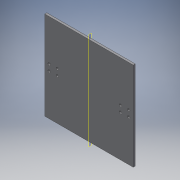
# Autodesk Inventor part: Hotplate
Saved by Autodesk Inventor 2019 (Build 230136000, 136)
## iProperties
Created: 2018-10-03
Part Number: Hotplate
Material: Generic
Document SubType Name: Modeling
Designer: LillaHunden
Mass: 231.125 g
Surface Area: 967.5 cm^2
Volume: 231.125 cm^3
Density: 1 g/cm^3
Appearance: Default
Author: LillaHunden
Autodesk Inventor part; units mm, degrees
ref_plane "YZ Plane" through (0, 0, 0) normal (1, 0, 0) x (0, 1, 0)
ref_plane "XZ Plane" through (0, 0, 0) normal (0, 1, 0) x (-1, 0, 0)
ref_plane "XY Plane" through (0, 0, 0) normal (0, 0, 1) x (1, 0, 0)
sketch "Sketch1" plane through (0, 0, 0) normal (0, 0, 1) x (1, 0, 0)
  line L0 (-107.5, -107.5) -> (107.5, -107.5)
  line L1 (107.5, -107.5) -> (107.5, 107.5)
  line L2 (107.5, 107.5) -> (-107.5, 107.5)
  line L3 (-107.5, 107.5) -> (-107.5, -107.5)
  line L4 (-107.5, -107.5) -> (107.5, 107.5) construction
  line L5 (107.5, -107.5) -> (-107.5, 107.5) construction
  point P0 (0, 0)
  dimension "d0" = 215
  dimension "d1" = 215
  constraints: 12 end point, 2 midpoint, 2 parallel, 1 horizontal, 1 perpendicular
  measures "d0" distance of L2.end L1.end
  measures "d1" distance of L1.end L0.end
extrude "Extrusion1" add sketch "Sketch1" along normal blind 5
ref_plane "Work Plane1" through (0, -107.5, 0) normal (-1, 0, 0) x (0, 0, 1)
sketch "Sketch3" plane through (0, 0, 5) normal (0, 0, 1) x (1, 0, 0)
  point P0 (96.652, 7.5)
  point P1 (96.652, -7.5)
  point P2 (76.652, -7.5)
  point P3 (76.652, 7.5)
  point P4 (-96.652, 7.5)
  point P5 (-76.652, 7.5)
  point P6 (-76.652, -7.5)
  point P7 (-96.652, -7.5)
hole "Hole1" at (96.652, 7.5, 5) at (96.652, -7.5, 5) at (76.652, -7.5, 5) at (76.652, 7.5, 5) at (-96.652, 7.5, 5) at (-76.652, 7.5, 5) at (-76.652, -7.5, 5) at (-96.652, -7.5, 5) direction (0, 0, -1) diameter 3.4 depth 5 countersink diameter 6.3 countersink angle 90
body "Solid1"
